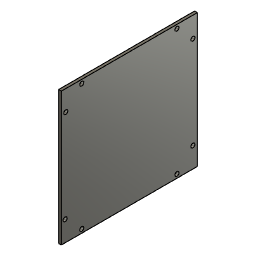
Сборка Cubesat 2.0 v6 (Autodesk Fusion 360 archive; units mm, degrees)
design "Боковые стенки Cubesat"
Autodesk Fusion 360 part; units mm, degrees
sketch "Sketch1" plane through (0, 0, 0) normal (1, 0, 0) x (0, 0, -1)
  line L0 (0, 0) -> (-100, 0)
  line L1 (-100, 0) -> (-100, 98)
  line L2 (-100, 98) -> (0, 98)
  line L3 (0, 98) -> (0, 0)
  dimension "d1" = 100
  dimension "d2" = 98
  constraint horizontal L0
  constraint vertical L1
  constraint horizontal L2
  constraint vertical L3
  constraint coincident L0.start L3.end
  measures "d1" distance of L0.start L0.end
  measures "d2" distance of L0.start L2.end
extrude "Extrude1" add sketch "Sketch1" against normal blind 2
extrude "Extrude2" add 1 faces at (0, 32.6667, 33.3333) along direction (1, 0, 0) blind 2
extrude "Extrude3" add 1 faces at (2, 32.6667, 33.3333) along direction (1, 0, 0) blind 1
sketch "Sketch2" plane through (3, 0, 0) normal (1, 0, 0) x (0, 0, -1)
  line L0 (-100, 98) -> (0, 98)
  line L1 (0, 98) -> (0, 0)
  line L2 (0, 0) -> (-100, 0)
  line L3 (-100, 0) -> (-100, 98)
  line L4 (-100, 98) -> (-85, 98)
  line L5 (-85, 98) -> (-85, 92.5)
  line L6 (-85, 92.5) -> (-100, 92.5)
  line L7 (-100, 92.5) -> (-100, 98)
  line L8 (-100, 98) -> (-93.5, 98)
  line L9 (-93.5, 98) -> (-93.5, 83)
  line L10 (0, 98) -> (-6.5, 98)
  line L11 (-6.5, 98) -> (-6.5, 83)
  line L12 (-6.5, 83) -> (0, 83)
  line L13 (0, 83) -> (0, 98)
  line L14 (0, 98) -> (-15, 98)
  line L15 (-15, 98) -> (-15, 92.5)
  line L16 (-15, 92.5) -> (0, 92.5)
  line L17 (0, 92.5) -> (0, 98)
  line L18 (0, 0) -> (-6.5, 0)
  line L19 (-6.5, 0) -> (-6.5, 15)
  line L20 (-6.5, 15) -> (0, 15)
  line L21 (0, 15) -> (0, 0)
  line L22 (0, 0) -> (-15, 0)
  line L23 (-15, 0) -> (-15, 5.5)
  line L24 (-15, 5.5) -> (0, 5.5)
  line L25 (0, 5.5) -> (0, 0)
  line L26 (-100, 0) -> (-85, 0)
  line L27 (-85, 0) -> (-85, 5.5)
  line L28 (-85, 5.5) -> (-100, 5.5)
  line L29 (-100, 5.5) -> (-100, 0)
  line L30 (-100, 0) -> (-94.5, 0)
  line L31 (-94.5, 0) -> (-94.5, 15)
  line L32 (-94.5, 15) -> (-100, 15)
  line L33 (-100, 15) -> (-100, 0)
  circle A0 centre (-85, 95.25) radius 1.5
  circle A1 centre (-97.25, 15) radius 1.5
  circle A2 centre (-85, 2.75) radius 1.5
  circle A3 centre (-15, 2.75) radius 1.5
  circle A4 centre (-3.25, 15) radius 1.5
  circle A5 centre (-3.25, 83) radius 1.5
  circle A6 centre (-15, 95.25) radius 1.5
  line L34 (-93.5, 83) -> (-100, 83)
  line L35 (-100, 83) -> (-100, 98)
  line L36 (-100, 98) -> (-93.5, 98)
  line L37 (-93.5, 98) -> (-93.5, 83)
  circle A7 centre (-96.75, 83) radius 1.5
  dimension "d53" = 15
  dimension "d54" = 5.5
  dimension "d55" = 6.5
  dimension "d57" = 6.5
  dimension "d58" = 15
  dimension "d59" = 15
  dimension "d60" = 5.5
  dimension "d61" = 6.5
  dimension "d62" = 15
  dimension "d63" = 5.5
  dimension "d64" = 15
  dimension "d65" = 5.5
  dimension "d66" = 15
  dimension "d67" = 100
  dimension "d68" = 98
  dimension "d69" = 5.5
  dimension "d70" = 15
  dimension "d71" = 3
  dimension "d73" = 3
  dimension "d74" = 3
  dimension "d75" = 3
  dimension "d76" = 3
  dimension "d77" = 3
  dimension "d78" = 3
  dimension "d81" = 15
  dimension "d83" = 3
  constraint horizontal L0
  constraint vertical L1
  constraint horizontal L2
  constraint vertical L3
  constraint coincident L1.end L2.start
  constraint horizontal L4
  constraint vertical L5
  constraint horizontal L6
  constraint vertical L7
  constraint horizontal L8
  constraint vertical L9
  constraint horizontal L10
  constraint vertical L11
  constraint horizontal L12
  constraint vertical L13
  constraint horizontal L14
  constraint vertical L15
  constraint horizontal L16
  constraint vertical L17
  constraint horizontal L18
  constraint vertical L19
  constraint horizontal L20
  constraint vertical L21
  constraint horizontal L22
  constraint vertical L23
  constraint horizontal L24
  constraint vertical L25
  constraint horizontal L26
  constraint vertical L27
  constraint horizontal L28
  constraint vertical L29
  constraint horizontal L30
  constraint vertical L31
  constraint horizontal L32
  constraint vertical L33
  constraint midpoint L5 A0.centre
  constraint midpoint L32 A1.centre
  constraint midpoint L27 A2.centre
  constraint midpoint L23 A3.centre
  constraint midpoint L20 A4.centre
  constraint midpoint L12 A5.centre
  constraint midpoint L15 A6.centre
  constraint horizontal L34
  constraint vertical L35
  constraint horizontal L36
  constraint vertical L37
  constraint midpoint L34 A7.centre
  measures "d53" distance of L0.start L4.end
  measures "d54" distance of L0.start L6.end
  measures "d55" distance of L0.start L8.end
  measures "d57" distance of L0.end L10.end
  measures "d58" distance of L0.end L12.end
  measures "d59" distance of L0.end L14.end
  measures "d60" distance of L0.end L16.end
  measures "d61" distance of L1.end L18.end
  measures "d62" distance of L1.end L20.end
  measures "d63" distance of L1.end L24.end
  measures "d64" distance of L2.end L26.end
  measures "d65" distance of L2.end L30.end
  measures "d66" distance of L2.end L32.end
  measures "d67" distance of L3 L13
  measures "d68" distance of L0 L2
  measures "d69" distance of L26 L28
  measures "d70" distance of L23 L25
  measures "d71" diameter of A0
  measures "d73" diameter of A1
  measures "d74" diameter of A2
  measures "d75" diameter of A3
  measures "d76" diameter of A4
  measures "d77" diameter of A5
  measures "d78" diameter of A6
  measures "d81" distance of L8 L34
  measures "d83" diameter of A7
extrude "Extrude9" cut sketch "Sketch2" against normal blind 20 contours L5 A0 | L5 A0 | L34 A7 | L34 A7 | L15 A6 | L15 A6 | L32 A1 | L32 A1 | L12 A5 | L12 A5 | L27 A2 | L27 A2 | L20 A4 | L20 A4 | L23 A3 | L23 A3
extrude "Extrude10" cut sketch "Sketch2" against normal blind 3 contours L0 L3 L4 L6 L7 L8 L9 L35 L36 L37 | L0 L4 L5 L6 L9 A0 L37 | L3 L6 L9 L34 L35 L37 A7 | L0 L1 L2 L3 L5 L6 L9 L11 L12 L15 L16 L19 L20 L23 L24 L27 L28 L31 L32 A0 A1 A2 A3 A4 A5 A6 L34 L37 A7 | L0 L11 L14 L15 L16 A6 | L3 L28 L31 L32 L33 A1 | L0 L1 L10 L11 L13 L14 L16 L17 | L2 L3 L26 L28 L29 L30 L31 L33 | L1 L11 L12 L13 L16 A5 | L2 L26 L27 L28 L31 A2 | L1 L19 L20 L21 L24 A4 | L2 L19 L22 L23 L24 A3 | L1 L2 L18 L19 L21 L22 L24 L25

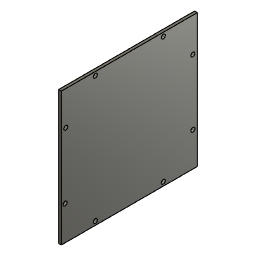
design "Боковые стенки Cubesat 2.0"
Autodesk Fusion 360 part; units mm, degrees
sketch "Sketch1" plane through (0, 0, 0) normal (1, 0, 0) x (0, 0, -1)
  line L0 (0, 0) -> (-100, 0)
  line L1 (-100, 0) -> (-100, 98)
  line L2 (-100, 98) -> (0, 98)
  line L3 (0, 98) -> (0, 0)
  dimension "d1" = 100
  dimension "d2" = 98
  constraint horizontal L0
  constraint vertical L1
  constraint horizontal L2
  constraint vertical L3
  constraint coincident L0.start L3.end
  measures "d1" distance of L0.start L0.end
  measures "d2" distance of L0.start L2.end
extrude "Extrude1" add sketch "Sketch1" against normal blind 2
extrude "Extrude2" add 1 faces at (0, 32.6667, 33.3333) along direction (1, 0, 0) blind 2
extrude "Extrude3" add 1 faces at (2, 32.6667, 33.3333) along direction (1, 0, 0) blind 1
sketch "Sketch2" plane through (3, 0, 0) normal (1, 0, 0) x (0, 0, -1)
  line L0 (-100, 98) -> (0, 98)
  line L1 (0, 98) -> (0, 0)
  line L2 (0, 0) -> (-100, 0)
  line L3 (-100, 0) -> (-100, 98)
  line L4 (-100, 98) -> (-75, 98)
  line L5 (-75, 98) -> (-75, 92.5)
  line L6 (-75, 92.5) -> (-100, 92.5)
  line L7 (-100, 92.5) -> (-100, 98)
  line L8 (-100, 98) -> (-93.5, 98)
  line L9 (-93.5, 98) -> (-93.5, 73)
  line L10 (0, 98) -> (-6.5, 98)
  line L11 (-6.5, 98) -> (-6.5, 73)
  line L12 (-6.5, 73) -> (0, 73)
  line L13 (0, 73) -> (0, 98)
  line L14 (0, 98) -> (-25, 98)
  line L15 (-25, 98) -> (-25, 92.5)
  line L16 (-25, 92.5) -> (0, 92.5)
  line L17 (0, 92.5) -> (0, 98)
  line L18 (0, 0) -> (-6.5, 0)
  line L19 (-6.5, 0) -> (-6.5, 25)
  line L20 (-6.5, 25) -> (0, 25)
  line L21 (0, 25) -> (0, 0)
  line L22 (0, 0) -> (-25, 0)
  line L23 (-25, 0) -> (-25, 5.5)
  line L24 (-25, 5.5) -> (0, 5.5)
  line L25 (0, 5.5) -> (0, 0)
  line L26 (-100, 0) -> (-75, 0)
  line L27 (-75, 0) -> (-75, 5.5)
  line L28 (-75, 5.5) -> (-100, 5.5)
  line L29 (-100, 5.5) -> (-100, 0)
  line L30 (-100, 0) -> (-94.5, 0)
  line L31 (-94.5, 0) -> (-94.5, 25)
  line L32 (-94.5, 25) -> (-100, 25)
  line L33 (-100, 25) -> (-100, 0)
  circle A0 centre (-75, 95.25) radius 1.5
  circle A1 centre (-97.25, 25) radius 1.5
  circle A2 centre (-75, 2.75) radius 1.5
  circle A3 centre (-25, 2.75) radius 1.5
  circle A4 centre (-3.25, 25) radius 1.5
  circle A5 centre (-3.25, 73) radius 1.5
  circle A6 centre (-25, 95.25) radius 1.5
  line L34 (-93.5, 73) -> (-100, 73)
  line L35 (-100, 73) -> (-100, 98)
  line L36 (-100, 98) -> (-93.5, 98)
  line L37 (-93.5, 98) -> (-93.5, 73)
  circle A7 centre (-96.75, 73) radius 1.5
  dimension "d53" = 25
  dimension "d54" = 5.5
  dimension "d55" = 6.5
  dimension "d57" = 6.5
  dimension "d58" = 25
  dimension "d59" = 25
  dimension "d60" = 5.5
  dimension "d61" = 6.5
  dimension "d62" = 25
  dimension "d63" = 5.5
  dimension "d64" = 25
  dimension "d65" = 5.5
  dimension "d66" = 25
  dimension "d67" = 100
  dimension "d68" = 98
  dimension "d69" = 5.5
  dimension "d70" = 25
  dimension "d71" = 3
  dimension "d73" = 3
  dimension "d74" = 3
  dimension "d75" = 3
  dimension "d76" = 3
  dimension "d77" = 3
  dimension "d78" = 3
  dimension "d81" = 25
  dimension "d83" = 3
  constraint horizontal L0
  constraint vertical L1
  constraint horizontal L2
  constraint vertical L3
  constraint coincident L1.end L2.start
  constraint horizontal L4
  constraint vertical L5
  constraint horizontal L6
  constraint vertical L7
  constraint horizontal L8
  constraint vertical L9
  constraint horizontal L10
  constraint vertical L11
  constraint horizontal L12
  constraint vertical L13
  constraint horizontal L14
  constraint vertical L15
  constraint horizontal L16
  constraint vertical L17
  constraint horizontal L18
  constraint vertical L19
  constraint horizontal L20
  constraint vertical L21
  constraint horizontal L22
  constraint vertical L23
  constraint horizontal L24
  constraint vertical L25
  constraint horizontal L26
  constraint vertical L27
  constraint horizontal L28
  constraint vertical L29
  constraint horizontal L30
  constraint vertical L31
  constraint horizontal L32
  constraint vertical L33
  constraint midpoint L5 A0.centre
  constraint midpoint L32 A1.centre
  constraint midpoint L27 A2.centre
  constraint midpoint L23 A3.centre
  constraint midpoint L20 A4.centre
  constraint midpoint L12 A5.centre
  constraint midpoint L15 A6.centre
  constraint horizontal L34
  constraint vertical L35
  constraint horizontal L36
  constraint vertical L37
  constraint midpoint L34 A7.centre
  measures "d53" distance of L0.start L4.end
  measures "d54" distance of L0.start L6.end
  measures "d55" distance of L0.start L8.end
  measures "d57" distance of L0.end L10.end
  measures "d58" distance of L0.end L12.end
  measures "d59" distance of L0.end L14.end
  measures "d60" distance of L0.end L16.end
  measures "d61" distance of L1.end L18.end
  measures "d62" distance of L1.end L20.end
  measures "d63" distance of L1.end L24.end
  measures "d64" distance of L2.end L26.end
  measures "d65" distance of L2.end L30.end
  measures "d66" distance of L2.end L32.end
  measures "d67" distance of L3 L13
  measures "d68" distance of L0 L2
  measures "d69" distance of L26 L28
  measures "d70" distance of L23 L25
  measures "d71" diameter of A0
  measures "d73" diameter of A1
  measures "d74" diameter of A2
  measures "d75" diameter of A3
  measures "d76" diameter of A4
  measures "d77" diameter of A5
  measures "d78" diameter of A6
  measures "d81" distance of L8 L34
  measures "d83" diameter of A7
extrude "Extrude9" cut sketch "Sketch2" against normal blind 20 contours L5 A0 | L5 A0 | L34 A7 | L34 A7 | L15 A6 | L15 A6 | L32 A1 | L32 A1 | L12 A5 | L12 A5 | L27 A2 | L27 A2 | L20 A4 | L20 A4 | L23 A3 | L23 A3
extrude "Extrude10" cut sketch "Sketch2" against normal blind 3 contours L0 L3 L4 L6 L7 L8 L9 L35 L36 L37 | L0 L4 L5 L6 L9 A0 L37 | L3 L6 L9 L34 L35 L37 A7 | L0 L1 L2 L3 L5 L6 L9 L11 L12 L15 L16 L19 L20 L23 L24 L27 L28 L31 L32 A0 A1 A2 A3 A4 A5 A6 L34 L37 A7 | L0 L11 L14 L15 L16 A6 | L3 L28 L31 L32 L33 A1 | L0 L1 L10 L11 L13 L14 L16 L17 | L2 L3 L26 L28 L29 L30 L31 L33 | L1 L11 L12 L13 L16 A5 | L2 L26 L27 L28 L31 A2 | L1 L19 L20 L21 L24 A4 | L2 L19 L22 L23 L24 A3 | L1 L2 L18 L19 L21 L22 L24 L25

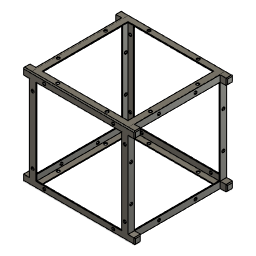
design "Cubesat 2.0"
Autodesk Fusion 360 part; units mm, degrees
sketch "Sketch1" plane through (0, 0, 0) normal (1, 0, 0) x (0, 0, -1)
  line L0 (0, 0) -> (-100, 0)
  line L1 (-100, 0) -> (-100, 100)
  line L2 (-100, 100) -> (0, 100)
  line L3 (0, 100) -> (0, 0)
  line L4 (-100, 100) -> (-93.5, 100)
  line L5 (-93.5, 100) -> (-93.5, 93.5)
  line L6 (-93.5, 93.5) -> (-100, 93.5)
  line L7 (-100, 93.5) -> (-100, 100)
  line L8 (0, 100) -> (-6.5, 100)
  line L9 (-6.5, 100) -> (-6.5, 93.5)
  line L10 (-6.5, 93.5) -> (0, 93.5)
  line L11 (0, 93.5) -> (0, 100)
  line L12 (-100, 0) -> (-93.5, 0)
  line L13 (-93.5, 0) -> (-93.5, 6.5)
  line L14 (-93.5, 6.5) -> (-100, 6.5)
  line L15 (-100, 6.5) -> (-100, 0)
  line L16 (0, 0) -> (-6.5, 0)
  line L17 (-6.5, 0) -> (-6.5, 6.5)
  line L18 (-6.5, 6.5) -> (0, 6.5)
  line L19 (0, 6.5) -> (0, 0)
  line L20 (-93.5, 93.5) -> (-6.5, 93.5)
  line L21 (-6.5, 93.5) -> (-6.5, 6.5)
  line L22 (-6.5, 6.5) -> (-93.5, 6.5)
  line L23 (-93.5, 6.5) -> (-93.5, 93.5)
  dimension "d1" = 100
  dimension "d2" = 100
  dimension "d3" = 6.5
  dimension "d4" = 6.5
  dimension "d5" = 6.5
  dimension "d6" = 6.5
  dimension "d7" = 6.5
  dimension "d8" = 6.5
  dimension "d9" = 6.5
  dimension "d10" = 6.5
  constraint horizontal L0
  constraint vertical L1
  constraint horizontal L2
  constraint vertical L3
  constraint coincident L0.start L3.end
  constraint horizontal L4
  constraint vertical L5
  constraint horizontal L6
  constraint vertical L7
  constraint horizontal L8
  constraint vertical L9
  constraint horizontal L10
  constraint vertical L11
  constraint horizontal L12
  constraint vertical L13
  constraint horizontal L14
  constraint vertical L15
  constraint horizontal L16
  constraint vertical L17
  constraint horizontal L18
  constraint vertical L19
  constraint horizontal L20
  constraint vertical L21
  constraint horizontal L22
  constraint vertical L23
  measures "d1" distance of L0.start L0.end
  measures "d2" distance of L0.start L2.end
  measures "d3" distance of L1.end L4.end
  measures "d4" distance of L1.end L6.end
  measures "d5" distance of L2.end L8.end
  measures "d6" distance of L2.end L10.end
  measures "d7" distance of L0.end L12.end
  measures "d8" distance of L0.end L14.end
  measures "d9" distance of L0.start L16.end
  measures "d10" distance of L0.start L18.end
extrude "Extrude1" add sketch "Sketch1" along normal blind 50 and the other way blind 50 contours L0 L3 L16 L17 L18 L19 | L0 L13 L17 L22 | L3 L10 L18 L21 | L0 L1 L12 L13 L14 L15 | L2 L3 L8 L9 L10 L11 | L1 L6 L14 L23 | L2 L5 L9 L20 | L1 L2 L4 L5 L6 L7
extrude "Extrude2" add sketch "Sketch1" along normal mid plane 113.5 contours L0 L3 L16 L17 L18 L19 | L0 L1 L12 L13 L14 L15 | L2 L3 L8 L9 L10 L11 | L1 L2 L4 L5 L6 L7
ref_plane "WorkPlane1" through (0, 50, 50) normal (0, 1, 0) x (0, 0, 1)
sketch "Sketch2" plane through (0, 50, 50) normal (0, 1, 0) x (1, 0, 0)
  line L0 (-50, -50) -> (50, -50)
  line L1 (50, -50) -> (50, 50)
  line L2 (50, 50) -> (-50, 50)
  line L3 (-50, 50) -> (-50, -50)
  line L4 (43.5, 43.5) -> (-43.5, 43.5)
  line L5 (-43.5, 43.5) -> (-43.5, -43.5)
  line L6 (-43.5, -43.5) -> (43.5, -43.5)
  line L7 (43.5, -43.5) -> (43.5, 43.5)
  line L8 (43.5, 43.5) -> (-43.5, -43.5) construction
  line L9 (-43.5, 43.5) -> (43.5, -43.5) construction
  dimension "d18" = 87
  dimension "d19" = 87
  dimension "d76" = 100
  dimension "d77" = 100
  dimension "d78" = 6.5
  dimension "d79" = 6.5
  constraint horizontal L0
  constraint vertical L1
  constraint horizontal L2
  constraint vertical L3
  constraint horizontal L4
  constraint perpendicular L4 L5
  constraint parallel L4 L6
  constraint parallel L5 L7
  constraint coincident L8 origin
  constraint coincident L9 origin
  measures "d18" distance of L5.end L6.end
  measures "d19" distance of L4.end L5.end
  measures "d76" distance of L1 L3
  measures "d77" distance of L0 L2
  measures "d78" distance of L1 L7
  measures "d79" distance of L0 L6
extrude "Extrude3" cut sketch "Sketch2" along normal mid plane 110 contours L4 L5 L6 L7
ref_plane "WorkPlane2" through (0, 50, 50) normal (0, 0, -1) x (0, 1, 0)
sketch "Sketch3" plane through (0, 50, 50) normal (0, 0, -1) x (1, 0, 0)
  line L0 (50, -50) -> (-50, -50)
  line L1 (-50, -50) -> (-50, 50)
  line L2 (-50, 50) -> (50, 50)
  line L3 (50, 50) -> (50, -50)
  line L4 (43.5, -43.5) -> (-43.5, -43.5)
  line L5 (-43.5, -43.5) -> (-43.5, 43.5)
  line L6 (-43.5, 43.5) -> (43.5, 43.5)
  line L7 (43.5, 43.5) -> (43.5, -43.5)
  line L8 (43.5, -43.5) -> (-43.5, 43.5) construction
  line L9 (-43.5, -43.5) -> (43.5, 43.5) construction
  dimension "d23" = 87
  dimension "d24" = 87
  dimension "d80" = 6.5
  dimension "d81" = 6.5
  dimension "d82" = 6.5
  dimension "d83" = 6.5
  constraint horizontal L0
  constraint vertical L1
  constraint horizontal L2
  constraint vertical L3
  constraint horizontal L4
  constraint perpendicular L4 L5
  constraint parallel L4 L6
  constraint parallel L5 L7
  constraint coincident L8 origin
  constraint coincident L9 origin
  measures "d23" distance of L5.end L6.end
  measures "d24" distance of L4.end L5.end
  measures "d80" distance of L2 L6
  measures "d81" distance of L1 L5
  measures "d82" distance of L3 L7
  measures "d83" distance of L0 L4
extrude "Extrude4" cut sketch "Sketch3" along normal mid plane 160 contours L4 L5 L6 L7
chamfer "Chamfer1" distance 0.8 angle 45 32 edges at (56.75, 100, 96.75) (56.75, 96.75, 100) (56.75, 96.75, 93.5) (56.75, 93.5, 96.75) (56.75, 6.5, 96.75) (56.75, 3.25, 93.5) (56.75, 0, 96.75) (56.75, 3.25, 100) (56.75, 0, 3.25) (56.75, 3.25, 6.5) (56.75, 6.5, 3.25) (56.75, 3.25, 0) (56.75, 100, 3.25) (56.75, 96.75, 6.5) (56.75, 93.5, 3.25) (56.75, 96.75, 0) (-56.75, 96.75, 0) (-56.75, 100, 3.25) (-56.75, 96.75, 6.5) (-56.75, 93.5, 3.25) (-56.75, 6.5, 3.25) (-56.75, 3.25, 0) (-56.75, 0, 3.25) (-56.75, 3.25, 6.5) (-56.75, 6.5, 96.75) (-56.75, 3.25, 93.5) (-56.75, 0, 96.75) (-56.75, 3.25, 100) (-56.75, 96.75, 93.5) (-56.75, 100, 96.75) (-56.75, 96.75, 100) (-56.75, 93.5, 96.75)
fillet "Fillet1" radius 1 4 edges at (0, 100, 100) (0, 100, 0) (0, 0, 100) (0, 0, 0)
ref_plane "WorkPlane3" through (0, 96.75, 3.25) normal (-1, 0, 0) x (0, 0, 1)
sketch "Sketch4" plane through (0, 96.75, 3.25) normal (-1, 0, 0) x (0, 0, -1)
  line L0 (2.45, 91.05) -> (-2.45, 91.05) construction
  line L1 (-2.45, 91.05) -> (-2.45, 95.95) construction
  line L2 (-2.45, 95.95) -> (2.45, 95.95) construction
  line L3 (2.45, 95.95) -> (2.45, 91.05) construction
  line L4 (-95.95, 95.95) -> (-91.05, 95.95) construction
  line L5 (-91.05, 95.95) -> (-91.05, 91.05) construction
  line L6 (-91.05, 91.05) -> (-95.95, 91.05) construction
  line L7 (-95.95, 91.05) -> (-95.95, 95.95) construction
  line L8 (-95.95, 2.45) -> (-91.05, 2.45) construction
  line L9 (-91.05, 2.45) -> (-91.05, -2.45) construction
  line L10 (-91.05, -2.45) -> (-95.95, -2.45) construction
  line L11 (-95.95, -2.45) -> (-95.95, 2.45) construction
  line L12 (-2.45, 2.45) -> (2.45, 2.45) construction
  line L13 (2.45, 2.45) -> (2.45, -2.45) construction
  line L14 (2.45, -2.45) -> (-2.45, -2.45) construction
  line L15 (-2.45, -2.45) -> (-2.45, 2.45) construction
  line L16 (2.45, 95.95) -> (-2.45, 91.05) construction
  line L17 (2.45, 91.05) -> (-2.45, 95.95) construction
  line L18 (-91.05, 2.45) -> (-95.95, -2.45) construction
  line L19 (-91.05, -2.45) -> (-95.95, 2.45) construction
  line L20 (0, 93.5) -> (-93.5, 93.5)
  line L21 (-93.5, 93.5) -> (-93.5, 0)
  line L22 (-93.5, 0) -> (0, 0)
  line L23 (0, 0) -> (0, 93.5)
  constraint coincident L2.end L3.start
  constraint coincident L0.end L1.start
  constraint coincident L0.start L3.end
  constraint coincident L1.end L2.start
  constraint coincident L8.end L9.start
  constraint coincident L10.end L11.start
  constraint coincident L9.end L10.start
  constraint coincident L8.start L11.end
  constraint horizontal L20
  constraint vertical L21
  constraint horizontal L22
  constraint vertical L23
  constraint midpoint L18 L21.end
  constraint midpoint L17 L20.start
extrude "Extrude5" cut sketch "Sketch4" along normal mid plane 98
sketch "Sketch5" plane through (0, 0, 3.25) normal (0, 0, 1) x (1, 0, 0)
  line L0 (43.5, 6.5) -> (-43.5, 6.5)
  line L1 (-43.5, 6.5) -> (-43.5, 93.5)
  line L2 (-43.5, 93.5) -> (43.5, 93.5)
  line L3 (43.5, 93.5) -> (43.5, 6.5)
  line L4 (-49, 3.25) -> (49, 3.25)
  line L5 (49, 3.25) -> (49, 96.75)
  line L6 (49, 96.75) -> (-49, 96.75)
  line L7 (-49, 96.75) -> (-49, 3.25)
  line L8 (49, 0.75) -> (-49, 0.75)
  line L9 (49, 0.75) -> (49, 99.25)
  line L10 (49, 99.25) -> (-49, 99.25)
  line L11 (-49, 99.25) -> (-49, 0.75)
  dimension "d32" = 2.5
  dimension "d33" = 2.5
  constraint perpendicular L7 L8
  constraint perpendicular L8 L9
  constraint perpendicular L9 L10
  constraint coincident L5 L8.start
  constraint coincident L6.end L11
  constraint vertical L11
  measures "d32" distance of L4 L8
  measures "d33" distance of L6 L10
extrude "Extrude6" cut sketch "Sketch5" along normal blind 95.75 and the other way blind 2.25
sketch "Sketch6" plane through (0, 0, 0) normal (1, 0, 0) x (0, 0, -1)
sketch "Sketch7" plane through (50, 0, 0) normal (1, 0, 0) x (0, 0, -1)
  line L0 (-6.5, 93.5) -> (-6.5, 100)
  line L1 (-6.5, 100) -> (-93.5, 100)
  line L2 (-93.5, 100) -> (-93.5, 93.5)
  line L3 (-93.5, 93.5) -> (-6.5, 93.5)
  line L4 (-93.5, 100) -> (-68.5, 100)
  line L5 (-68.5, 100) -> (-68.5, 93.5)
  line L6 (-68.5, 93.5) -> (-93.5, 93.5)
  line L7 (-93.5, 93.5) -> (-93.5, 100)
  line L8 (-6.5, 100) -> (-31.5, 100)
  line L9 (-31.5, 100) -> (-31.5, 93.5)
  line L10 (-31.5, 93.5) -> (-6.5, 93.5)
  line L11 (-6.5, 93.5) -> (-6.5, 100)
  circle A0 centre (-68.5, 96.75) radius 1.5
  circle A1 centre (-31.5, 96.75) radius 1.5
  line L12 (-93.5, 93.5) -> (-100, 93.5)
  line L13 (-100, 93.5) -> (-100, 6.5)
  line L14 (-100, 6.5) -> (-93.5, 6.5)
  line L15 (-93.5, 6.5) -> (-93.5, 93.5)
  line L16 (-100, 6.5) -> (-93.5, 6.5)
  line L17 (-93.5, 6.5) -> (-93.5, 31.5)
  line L18 (-93.5, 31.5) -> (-100, 31.5)
  line L19 (-100, 31.5) -> (-100, 6.5)
  line L20 (-100, 93.5) -> (-93.5, 93.5)
  line L21 (-93.5, 93.5) -> (-93.5, 68.5)
  line L22 (-93.5, 68.5) -> (-100, 68.5)
  line L23 (-100, 68.5) -> (-100, 93.5)
  line L24 (-93.5, 6.5) -> (-68.5, 6.5)
  line L25 (-68.5, 6.5) -> (-68.5, 0)
  line L26 (-68.5, 0) -> (-93.5, 0)
  line L27 (-93.5, 0) -> (-93.5, 6.5)
  line L28 (-6.4996, 6.5) -> (-31.4996, 6.5)
  line L29 (-31.4996, 6.5) -> (-31.4996, 0)
  line L30 (-31.4996, 0) -> (-6.4996, 0)
  line L31 (-6.4996, 0) -> (-6.4996, 6.5)
  line L32 (-6.4996, 6.5) -> (0, 6.5)
  line L33 (0, 6.5) -> (0, 31.5)
  line L34 (0, 31.5) -> (-6.4996, 31.5)
  line L35 (-6.4996, 31.5) -> (-6.4996, 6.5)
  line L36 (-6.5, 93.5) -> (0, 93.5)
  line L37 (0, 93.5) -> (0, 68.5)
  line L38 (0, 68.5) -> (-6.5, 68.5)
  line L39 (-6.5, 68.5) -> (-6.5, 93.5)
  circle A2 centre (-96.75, 68.5) radius 1.5
  circle A3 centre (-96.75, 31.5) radius 1.5
  circle A4 centre (-68.5, 3.25) radius 1.5
  circle A5 centre (-31.4996, 3.25) radius 1.5
  circle A6 centre (-3.2498, 31.5) radius 1.5
  circle A7 centre (-3.25, 68.5) radius 1.5
  point P0 (-100, 93.5)
  point P1 (-6.5, 6.5)
  dimension "d36" = 25
  dimension "d37" = 25
  dimension "d38" = 3
  dimension "d39" = 3
  dimension "d40" = 3.25
  dimension "d41" = 3.25
  dimension "d42" = 25
  dimension "d43" = 25
  dimension "d44" = 25
  dimension "d45" = 25
  dimension "d46" = 25
  dimension "d47" = 6.5
  dimension "d48" = 25
  dimension "d49" = 3
  dimension "d50" = 3
  dimension "d51" = 3
  dimension "d52" = 3
  dimension "d53" = 3
  dimension "d54" = 3
  dimension "d55" = 3.25
  dimension "d56" = 87
  dimension "d57" = 3.25
  dimension "d58" = 3.25
  dimension "d59" = 3.25
  dimension "d60" = 37.0004
  dimension "d61" = 3.2498
  constraint horizontal L4
  constraint vertical L5
  constraint horizontal L6
  constraint vertical L7
  constraint coincident L1.end L2.start
  constraint horizontal L8
  constraint vertical L9
  constraint horizontal L10
  constraint vertical L11
  constraint coincident L0.end L1.start
  constraint midpoint L5 A0.centre
  constraint midpoint L9 A1.centre
  constraint horizontal L12
  constraint vertical L13
  constraint horizontal L14
  constraint vertical L15
  constraint horizontal L16
  constraint vertical L17
  constraint horizontal L18
  constraint vertical L19
  constraint horizontal L20
  constraint vertical L21
  constraint horizontal L22
  constraint vertical L23
  constraint horizontal L24
  constraint vertical L25
  constraint horizontal L26
  constraint vertical L27
  constraint horizontal L28
  constraint vertical L29
  constraint horizontal L30
  constraint vertical L31
  constraint horizontal L32
  constraint vertical L33
  constraint horizontal L34
  constraint vertical L35
  constraint horizontal L36
  constraint vertical L37
  constraint horizontal L38
  constraint vertical L39
  constraint midpoint L22 A2.centre
  constraint midpoint L18 A3.centre
  constraint midpoint L25 A4.centre
  constraint midpoint L29 A5.centre
  constraint midpoint L34 A6.centre
  constraint midpoint L38 A7.centre
  constraint coincident L13 P0
  constraint coincident L28 P1
  measures "d36" distance of L1.end L4.end
  measures "d37" distance of L0.end L8.end
  measures "d38" diameter of A0
  measures "d39" diameter of A1
  measures "d40" distance of L4 A0.centre
  measures "d41" distance of L10 A1.centre
  measures "d42" distance of L13.end L18.end
  measures "d43" distance of P0 L22.end
  measures "d44" distance of L14.end L24.end
  measures "d45" distance of L28.start L28.end
  measures "d46" distance of L28.start L34.end
  measures "d47" distance of L0.start L36.end
  measures "d48" distance of L0.start L38.end
  measures "d49" diameter of A2
  measures "d50" diameter of A3
  measures "d51" diameter of A4
  measures "d52" diameter of A5
  measures "d53" diameter of A6
  measures "d54" diameter of A7
  measures "d55" distance of L21 A2.centre
  measures "d56" distance of P0 L13.end
  measures "d57" distance of L13 A3.centre
  measures "d58" distance of L24 A4.centre
  measures "d59" distance of L28 A5.centre
  measures "d60" distance of A4.centre A5.centre
  measures "d61" distance of L35 A6.centre
extrude "Extrude7" cut sketch "Sketch7" against normal blind 120 contours L9 A1 | L9 A1 | L38 A7 | L38 A7 | L5 A0 | L5 A0 | L22 A2 | L22 A2 | L18 A3 | L18 A3 | L25 A4 | L25 A4 | L29 A5 | L29 A5 | L34 A6 | L34 A6
sketch "Sketch8" plane through (0, 0, 0) normal (0, 0, -1) x (-1, 0, 0)
  line L0 (-55.95, 1) -> (55.95, 1)
  line L1 (55.95, 1) -> (55.95, 6.5)
  line L2 (55.95, 6.5) -> (50, 6.5)
  line L3 (50, 6.5) -> (50, 93.5)
  line L4 (50, 93.5) -> (55.95, 93.5)
  line L5 (55.95, 93.5) -> (55.95, 99)
  line L6 (55.95, 99) -> (-55.95, 99)
  line L7 (-55.95, 99) -> (-55.95, 93.5)
  line L8 (-55.95, 93.5) -> (-50, 93.5)
  line L9 (-50, 93.5) -> (-50, 6.5)
  line L10 (-50, 6.5) -> (-55.95, 6.5)
  line L11 (-55.95, 6.5) -> (-55.95, 1)
  line L12 (-43.5, 6.5) -> (-43.5, 93.5)
  line L13 (-43.5, 93.5) -> (43.5, 93.5)
  line L14 (43.5, 93.5) -> (43.5, 6.5)
  line L15 (43.5, 6.5) -> (-43.5, 6.5)
  line L16 (-50, 93.5) -> (-35, 93.5)
  line L17 (-35, 93.5) -> (-35, 99)
  line L18 (-35, 99) -> (-50, 99)
  line L19 (-50, 99) -> (-50, 93.5)
  line L20 (-50, 99) -> (-43.5, 99)
  line L21 (-43.5, 99) -> (-43.5, 84)
  line L22 (-43.5, 84) -> (-50, 84)
  line L23 (-50, 84) -> (-50, 99)
  line L24 (50, 93.5) -> (35, 93.5)
  line L25 (35, 93.5) -> (35, 99)
  line L26 (35, 99) -> (50, 99)
  line L27 (50, 99) -> (50, 93.5)
  line L28 (50, 99) -> (43.5, 99)
  line L29 (43.5, 99) -> (43.5, 84)
  line L30 (43.5, 84) -> (50, 84)
  line L31 (50, 84) -> (50, 99)
  line L32 (50, 6.5) -> (35, 6.5)
  line L33 (35, 6.5) -> (35, 1)
  line L34 (35, 1) -> (50, 1)
  line L35 (50, 1) -> (50, 6.5)
  line L36 (50, 1) -> (43.5, 1)
  line L37 (43.5, 1) -> (43.5, 16)
  line L38 (43.5, 16) -> (50, 16)
  line L39 (50, 16) -> (50, 1)
  line L40 (-50, 1) -> (-43.5, 1)
  line L41 (-43.5, 1) -> (-43.5, 16)
  line L42 (-43.5, 16) -> (-50, 16)
  line L43 (-50, 16) -> (-50, 1)
  line L44 (-50, 6.5) -> (-35, 6.5)
  line L45 (-35, 6.5) -> (-35, 1)
  line L46 (-35, 1) -> (-50, 1)
  line L47 (-50, 1) -> (-50, 6.5)
  circle A0 centre (35, 3.75) radius 1.5
  circle A1 centre (-35, 3.75) radius 1.5
  circle A2 centre (-46.75, 16) radius 1.5
  circle A3 centre (-46.75, 84) radius 1.5
  circle A4 centre (-35, 96.25) radius 1.5
  circle A5 centre (35, 96.25) radius 1.5
  circle A6 centre (46.75, 84) radius 1.5
  circle A7 centre (46.75, 16) radius 1.5
  dimension "d66" = 15
  dimension "d67" = 15
  dimension "d68" = 5.5
  dimension "d69" = 6.5
  dimension "d70" = 15
  dimension "d71" = 15
  dimension "d72" = 6.5
  dimension "d73" = 5.5
  dimension "d74" = 15
  dimension "d75" = 15
  dimension "d84" = 5.5
  dimension "d85" = 15
  dimension "d86" = 15
  dimension "d87" = 3
  dimension "d88" = 3
  dimension "d89" = 3
  dimension "d90" = 3
  dimension "d91" = 3
  dimension "d92" = 3
  dimension "d93" = 3
  dimension "d94" = 3
  dimension "d95" = 2.75
  dimension "d96" = 3.25
  dimension "d97" = 8.5
  constraint horizontal L16
  constraint vertical L17
  constraint horizontal L18
  constraint vertical L19
  constraint coincident L8.end L9.start
  constraint horizontal L20
  constraint vertical L21
  constraint horizontal L22
  constraint vertical L23
  constraint horizontal L24
  constraint vertical L25
  constraint horizontal L26
  constraint vertical L27
  constraint coincident L3.end L4.start
  constraint horizontal L28
  constraint vertical L29
  constraint horizontal L30
  constraint vertical L31
  constraint horizontal L32
  constraint vertical L33
  constraint horizontal L34
  constraint vertical L35
  constraint coincident L2.end L3.start
  constraint horizontal L36
  constraint vertical L37
  constraint horizontal L38
  constraint vertical L39
  constraint coincident L14 L37.end
  constraint horizontal L40
  constraint vertical L41
  constraint horizontal L42
  constraint vertical L43
  constraint coincident L0 L40.start
  constraint horizontal L44
  constraint vertical L45
  constraint horizontal L46
  constraint vertical L47
  constraint coincident L9.end L10.start
  constraint midpoint L33 A0.centre
  constraint midpoint L45 A1.centre
  constraint midpoint L42 A2.centre
  constraint midpoint L22 A3.centre
  constraint midpoint L17 A4.centre
  constraint midpoint L25 A5.centre
  constraint midpoint L30 A6.centre
  constraint midpoint L38 A7.centre
  measures "d66" distance of L8.end L16.end
  measures "d67" distance of L18.end L22.end
  measures "d68" distance of L16 L18
  measures "d69" distance of L19 L21
  measures "d70" distance of L3.end L24.end
  measures "d71" distance of L26.end L30.end
  measures "d72" distance of L29 L31
  measures "d73" distance of L24 L26
  measures "d74" distance of L2.end L32.end
  measures "d75" distance of L34.end L38.end
  measures "d84" distance of L32 L34
  measures "d85" distance of L40.start L42.end
  measures "d86" distance of L9.end L44.end
  measures "d87" diameter of A0
  measures "d88" diameter of A1
  measures "d89" diameter of A2
  measures "d90" diameter of A3
  measures "d91" diameter of A4
  measures "d92" diameter of A5
  measures "d93" diameter of A6
  measures "d94" diameter of A7
  measures "d95" distance of L46 A1.centre
  measures "d96" distance of L41 A2.centre
  measures "d97" distance of L41 A1.centre
extrude "Extrude8" cut sketch "Sketch8" against normal blind 160 contours L45 A1 | L45 A1 | L42 A2 | L42 A2 | L33 A0 | L33 A0 | L22 A3 | L22 A3 | L38 A7 | L38 A7 | L17 A4 | L17 A4 | L30 A6 | L30 A6 | L25 A5 | L25 A5
sketch "Sketch9" plane through (0, 0, 0) normal (0, 0, -1) x (-1, 0, 0)
  circle A0 centre (-46.75, 84) radius 1.5
  circle A1 centre (46.75, 16) radius 1.5
  circle A2 centre (46.75, 84) radius 1.5
  circle A3 centre (-46.75, 16) radius 1.5
  circle A4 centre (-35, 96.25) radius 1.5
  circle A5 centre (35, 3.75) radius 1.5
  circle A6 centre (35, 96.25) radius 1.5
  circle A7 centre (-35, 3.75) radius 1.5
  line L0 (-55.95, 1) -> (55.95, 1)
  line L1 (55.95, 1) -> (55.95, 6.5)
  line L2 (55.95, 6.5) -> (50, 6.5)
  line L3 (50, 6.5) -> (50, 93.5)
  line L4 (50, 93.5) -> (55.95, 93.5)
  line L5 (55.95, 93.5) -> (55.95, 99)
  line L6 (55.95, 99) -> (-55.95, 99)
  line L7 (-55.95, 99) -> (-55.95, 93.5)
  line L8 (-55.95, 93.5) -> (-50, 93.5)
  line L9 (-50, 93.5) -> (-50, 6.5)
  line L10 (-50, 6.5) -> (-55.95, 6.5)
  line L11 (-55.95, 6.5) -> (-55.95, 1)
  line L12 (-43.5, 6.5) -> (-43.5, 93.5)
  line L13 (-43.5, 93.5) -> (43.5, 93.5)
  line L14 (43.5, 93.5) -> (43.5, 6.5)
  line L15 (43.5, 6.5) -> (-43.5, 6.5)
sketch "Sketch11" plane through (0, 100, 0) normal (0, 1, 0) x (-1, 0, 0)
  line L0 (-43.5, 93.5) -> (43.5, 93.5)
  line L1 (43.5, 93.5) -> (43.5, 6.5)
  line L2 (43.5, 6.5) -> (-43.5, 6.5)
  line L3 (-43.5, 6.5) -> (-43.5, 93.5)
  line L4 (-55.95, 1) -> (55.95, 1)
  line L5 (55.95, 1) -> (55.95, 6.5)
  line L6 (55.95, 6.5) -> (50, 6.5)
  line L7 (50, 6.5) -> (50, 93.5)
  line L8 (50, 93.5) -> (55.95, 93.5)
  line L9 (55.95, 93.5) -> (55.95, 99)
  line L10 (55.95, 99) -> (-55.95, 99)
  line L11 (-55.95, 99) -> (-55.95, 93.5)
  line L12 (-55.95, 93.5) -> (-50, 93.5)
  line L13 (-50, 93.5) -> (-50, 6.5)
  line L14 (-50, 6.5) -> (-55.95, 6.5)
  line L15 (-55.95, 6.5) -> (-55.95, 1)
  line L16 (-50, 1) -> (50, 1)
  line L17 (50, 1) -> (50, 99)
  line L18 (50, 99) -> (-50, 99)
  line L19 (-50, 99) -> (-50, 1)
  line L20 (50, 1) -> (25, 1)
  line L21 (25, 1) -> (25, 6.5)
  line L22 (25, 6.5) -> (50, 6.5)
  line L23 (50, 6.5) -> (50, 1)
  line L24 (50, 1) -> (43.5, 1)
  line L25 (43.5, 1) -> (43.5, 26)
  line L26 (43.5, 26) -> (50, 26)
  line L27 (50, 26) -> (50, 1)
  line L28 (-50, 1) -> (-25, 1)
  line L29 (-25, 1) -> (-25, 6.5)
  line L30 (-25, 6.5) -> (-50, 6.5)
  line L31 (-50, 6.5) -> (-50, 1)
  line L32 (-50, 1) -> (-43.5, 1)
  line L33 (-43.5, 1) -> (-43.5, 26)
  line L34 (-43.5, 26) -> (-50, 26)
  line L35 (-50, 26) -> (-50, 1)
  line L36 (-50, 99) -> (-43.5, 99)
  line L37 (-43.5, 99) -> (-43.5, 74)
  line L38 (-43.5, 74) -> (-50, 74)
  line L39 (-50, 74) -> (-50, 99)
  line L40 (-50, 99) -> (-25, 99)
  line L41 (-25, 99) -> (-25, 93.5)
  line L42 (-25, 93.5) -> (-50, 93.5)
  line L43 (-50, 93.5) -> (-50, 99)
  line L44 (50, 99) -> (25, 99)
  line L45 (25, 99) -> (25, 93.5)
  line L46 (25, 93.5) -> (50, 93.5)
  line L47 (50, 93.5) -> (50, 99)
  line L48 (50, 99) -> (43.5, 99)
  line L49 (43.5, 99) -> (43.5, 74)
  line L50 (43.5, 74) -> (50, 74)
  line L51 (50, 74) -> (50, 99)
  circle A0 centre (25, 3.75) radius 1.5
  circle A1 centre (46.75, 26) radius 1.5
  circle A2 centre (-25, 3.75) radius 1.5
  circle A3 centre (-46.75, 26) radius 1.5
  circle A4 centre (-46.75, 74) radius 1.5
  circle A5 centre (-25, 96.25) radius 1.5
  circle A6 centre (25, 96.25) radius 1.5
  circle A7 centre (46.75, 74) radius 1.5
  dimension "d109" = 100
  dimension "d110" = 98
  dimension "d111" = 6.5
  dimension "d112" = 25
  dimension "d113" = 5.5
  dimension "d114" = 25
  dimension "d115" = 25
  dimension "d116" = 5.5
  dimension "d117" = 25
  dimension "d118" = 6.5
  dimension "d119" = 25
  dimension "d120" = 25
  dimension "d121" = 25
  dimension "d122" = 5.5
  dimension "d123" = 25
  dimension "d124" = 6.5
  dimension "d125" = 6.5
  dimension "d126" = 5.5
  dimension "d127" = 6.5
  dimension "d128" = 3
  dimension "d129" = 3
  dimension "d130" = 3
  dimension "d131" = 3
  dimension "d132" = 3
  dimension "d133" = 3
  dimension "d134" = 3
  dimension "d135" = 3
  constraint horizontal L16
  constraint vertical L17
  constraint horizontal L18
  constraint vertical L19
  constraint coincident L4 L16.start
  constraint horizontal L20
  constraint vertical L21
  constraint horizontal L22
  constraint vertical L23
  constraint horizontal L24
  constraint vertical L25
  constraint horizontal L26
  constraint vertical L27
  constraint horizontal L28
  constraint vertical L29
  constraint horizontal L30
  constraint vertical L31
  constraint horizontal L32
  constraint vertical L33
  constraint horizontal L34
  constraint vertical L35
  constraint horizontal L36
  constraint vertical L37
  constraint horizontal L38
  constraint vertical L39
  constraint horizontal L40
  constraint vertical L41
  constraint horizontal L42
  constraint vertical L43
  constraint horizontal L44
  constraint vertical L45
  constraint horizontal L46
  constraint vertical L47
  constraint horizontal L48
  constraint vertical L49
  constraint horizontal L50
  constraint vertical L51
  constraint midpoint L21 A0.centre
  constraint midpoint L26 A1.centre
  constraint midpoint L29 A2.centre
  constraint midpoint L34 A3.centre
  constraint midpoint L38 A4.centre
  constraint midpoint L41 A5.centre
  constraint midpoint L45 A6.centre
  constraint midpoint L50 A7.centre
  measures "d109" distance of L16.start L16.end
  measures "d110" distance of L16.start L18.end
  measures "d111" distance of L3 L19
  measures "d112" distance of L16.end L20.end
  measures "d113" distance of L16.end L6.end
  measures "d114" distance of L16.end L26.end
  measures "d115" distance of L16.start L28.end
  measures "d116" distance of L16.start L13.end
  measures "d117" distance of L16.start L34.end
  measures "d118" distance of L33.end L34.end
  measures "d119" distance of L18.end L38.end
  measures "d120" distance of L18.end L40.end
  measures "d121" distance of L17.end L44.end
  measures "d122" distance of L44.end L45.end
  measures "d123" distance of L17.end L50.end
  measures "d124" distance of L25 L27
  measures "d125" distance of L19 L37
  measures "d126" distance of L18 L42
  measures "d127" distance of L17 L49
  measures "d128" diameter of A0
  measures "d129" diameter of A1
  measures "d130" diameter of A2
  measures "d131" diameter of A3
  measures "d132" diameter of A4
  measures "d133" diameter of A5
  measures "d134" diameter of A6
  measures "d135" diameter of A7
extrude "Extrude9" cut sketch "Sketch11" against normal blind 120 contours L41 A5 | L41 A5 | L38 A4 | L38 A4 | L45 A6 | L45 A6 | L34 A3 | L34 A3 | L50 A7 | L50 A7 | L29 A2 | L29 A2 | L26 A1 | L26 A1 | L21 A0 | L21 A0

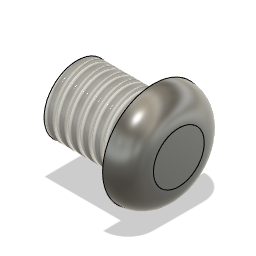
design "Болт M4"
Autodesk Fusion 360 part; units mm, degrees
sketch "Sketch1" plane through (0, 0, 0) normal (1, 0, 0) x (0, 0, -1)
  circle A0 centre (0, 0) radius 1.5
  dimension "d1" = 3
  constraint coincident A0.centre origin
  measures "d1" diameter of A0
extrude "Extrude1" add sketch "Sketch1" along normal blind 4.5
sketch "Sketch2" plane through (4.5, 0, 0) normal (1, 0, 0) x (0, 0, -1)
  circle A0 centre (0, 0) radius 1.5
  circle A1 centre (0, 0) radius 3
  dimension "d4" = 6
  constraint concentric A0 A1
  measures "d4" diameter of A1
extrude "Extrude2" add sketch "Sketch2" along normal blind 1.5 contours A0 | A1
fillet "Fillet1" radius 1.5 1 edges at (6, -1.0848, 2.797)
thread "Thread1" "ISO Metric profile 4.0 M4x0.7 6g" major diameter 3.908 minor diameter 3.111 pitch 0.7 angle 60 resizes the face on face at (3, -0.0748, -1.4981)

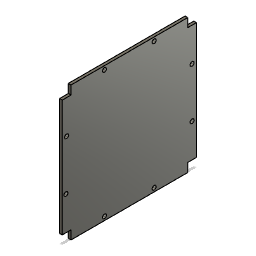
design "Боковые стенки Cubesatb 3.0"
Autodesk Fusion 360 part; units mm, degrees
sketch "Sketch1" plane through (0, 0, 0) normal (1, 0, 0) x (0, 0, -1)
  line L0 (0, 0) -> (-100, 0)
  line L1 (-100, 0) -> (-100, 100)
  line L2 (-100, 100) -> (0, 100)
  line L3 (0, 100) -> (0, 0)
  dimension "d1" = 100
  dimension "d2" = 100
  constraint horizontal L0
  constraint vertical L1
  constraint horizontal L2
  constraint vertical L3
  constraint coincident L0.start L3.end
  measures "d1" distance of L0.start L0.end
  measures "d2" distance of L0.start L2.end
extrude "Extrude1" add sketch "Sketch1" against normal blind 2
extrude "Extrude2" add 1 faces at (0, 33.3333, 33.3333) along direction (1, 0, 0) blind 2
extrude "Extrude3" add 1 faces at (2, 33.3333, 33.3333) along direction (1, 0, 0) blind 1
sketch "Sketch2" plane through (3, 0, 0) normal (1, 0, 0) x (0, 0, -1)
  line L0 (-100, 100) -> (0, 100)
  line L1 (0, 100) -> (0, 0)
  line L2 (0, 0) -> (-100, 0)
  line L3 (-100, 0) -> (-100, 100)
  line L4 (-100, 100) -> (-68.5, 100)
  line L5 (-68.5, 100) -> (-68.5, 94.5)
  line L6 (-68.5, 94.5) -> (-100, 94.5)
  line L7 (-100, 94.5) -> (-100, 100)
  line L8 (-100, 100) -> (-93.5, 100)
  line L9 (-93.5, 100) -> (-93.5, 68.5)
  line L10 (0, 100) -> (-6.5, 100)
  line L11 (-6.5, 100) -> (-6.5, 68.5)
  line L12 (-6.5, 68.5) -> (0, 68.5)
  line L13 (0, 68.5) -> (0, 100)
  line L14 (0, 100) -> (-31.5, 100)
  line L15 (-31.5, 100) -> (-31.5, 94.5)
  line L16 (-31.5, 94.5) -> (0, 94.5)
  line L17 (0, 94.5) -> (0, 100)
  line L18 (0, 0) -> (-6.5, 0)
  line L19 (-6.5, 0) -> (-6.5, 31.5)
  line L20 (-6.5, 31.5) -> (0, 31.5)
  line L21 (0, 31.5) -> (0, 0)
  line L22 (0, 0) -> (-31.5, 0)
  line L23 (-31.5, 0) -> (-31.5, 5.5)
  line L24 (-31.5, 5.5) -> (0, 5.5)
  line L25 (0, 5.5) -> (0, 0)
  line L26 (-100, 0) -> (-68.5, 0)
  line L27 (-68.5, 0) -> (-68.5, 5.5)
  line L28 (-68.5, 5.5) -> (-100, 5.5)
  line L29 (-100, 5.5) -> (-100, 0)
  line L30 (-100, 0) -> (-94.5, 0)
  line L31 (-94.5, 0) -> (-94.5, 31.5)
  line L32 (-94.5, 31.5) -> (-100, 31.5)
  line L33 (-100, 31.5) -> (-100, 0)
  circle A0 centre (-68.5, 97.25) radius 1.5
  circle A1 centre (-97.25, 31.5) radius 1.5
  circle A2 centre (-68.5, 2.75) radius 1.5
  circle A3 centre (-31.5, 2.75) radius 1.5
  circle A4 centre (-3.25, 31.5) radius 1.5
  circle A5 centre (-3.25, 68.5) radius 1.5
  circle A6 centre (-31.5, 97.25) radius 1.5
  line L34 (-93.5, 68.5) -> (-100, 68.5)
  line L35 (-100, 68.5) -> (-100, 100)
  line L36 (-100, 100) -> (-93.5, 100)
  line L37 (-93.5, 100) -> (-93.5, 68.5)
  circle A7 centre (-96.75, 68.5) radius 1.5
  line L38 (-100, 100) -> (-93.5, 100)
  line L39 (-93.5, 100) -> (-93.5, 93.5)
  line L40 (-93.5, 93.5) -> (-100, 93.5)
  line L41 (-100, 93.5) -> (-100, 100)
  line L42 (-100, 0) -> (-93.5, 0)
  line L43 (-93.5, 0) -> (-93.5, 6.5)
  line L44 (-93.5, 6.5) -> (-100, 6.5)
  line L45 (-100, 6.5) -> (-100, 0)
  line L46 (0, 0) -> (-6.5, 0)
  line L47 (-6.5, 0) -> (-6.5, 6.5)
  line L48 (-6.5, 6.5) -> (0, 6.5)
  line L49 (0, 6.5) -> (0, 0)
  line L50 (0, 100) -> (-6.5, 100)
  line L51 (-6.5, 100) -> (-6.5, 93.5)
  line L52 (-6.5, 93.5) -> (0, 93.5)
  line L53 (0, 93.5) -> (0, 100)
  dimension "d53" = 31.5
  dimension "d54" = 5.5
  dimension "d55" = 6.5
  dimension "d57" = 6.5
  dimension "d58" = 31.5
  dimension "d59" = 31.5
  dimension "d60" = 5.5
  dimension "d61" = 6.5
  dimension "d62" = 31.5
  dimension "d63" = 5.5
  dimension "d64" = 31.5
  dimension "d65" = 5.5
  dimension "d66" = 31.5
  dimension "d67" = 100
  dimension "d68" = 100
  dimension "d69" = 5.5
  dimension "d70" = 31.5
  dimension "d71" = 3
  dimension "d73" = 3
  dimension "d74" = 3
  dimension "d75" = 3
  dimension "d76" = 3
  dimension "d77" = 3
  dimension "d78" = 3
  dimension "d81" = 31.5
  dimension "d83" = 3
  dimension "d88" = 6.5
  dimension "d89" = 6.5
  dimension "d90" = 6.5
  dimension "d91" = 6.5
  dimension "d92" = 6.5
  dimension "d93" = 6.5
  dimension "d94" = 6.5
  dimension "d95" = 6.5
  constraint horizontal L0
  constraint vertical L1
  constraint horizontal L2
  constraint vertical L3
  constraint coincident L1.end L2.start
  constraint horizontal L4
  constraint vertical L5
  constraint horizontal L6
  constraint vertical L7
  constraint horizontal L8
  constraint vertical L9
  constraint horizontal L10
  constraint vertical L11
  constraint horizontal L12
  constraint vertical L13
  constraint horizontal L14
  constraint vertical L15
  constraint horizontal L16
  constraint vertical L17
  constraint horizontal L18
  constraint vertical L19
  constraint horizontal L20
  constraint vertical L21
  constraint horizontal L22
  constraint vertical L23
  constraint horizontal L24
  constraint vertical L25
  constraint horizontal L26
  constraint vertical L27
  constraint horizontal L28
  constraint vertical L29
  constraint horizontal L30
  constraint vertical L31
  constraint horizontal L32
  constraint vertical L33
  constraint midpoint L5 A0.centre
  constraint midpoint L32 A1.centre
  constraint midpoint L27 A2.centre
  constraint midpoint L23 A3.centre
  constraint midpoint L20 A4.centre
  constraint midpoint L12 A5.centre
  constraint midpoint L15 A6.centre
  constraint horizontal L34
  constraint vertical L35
  constraint horizontal L36
  constraint vertical L37
  constraint midpoint L34 A7.centre
  constraint horizontal L38
  constraint vertical L39
  constraint horizontal L40
  constraint vertical L41
  constraint horizontal L42
  constraint vertical L43
  constraint horizontal L44
  constraint vertical L45
  constraint horizontal L46
  constraint vertical L47
  constraint horizontal L48
  constraint vertical L49
  constraint horizontal L50
  constraint vertical L51
  constraint horizontal L52
  constraint vertical L53
  measures "d53" distance of L0.start L4.end
  measures "d54" distance of L0.start L6.end
  measures "d55" distance of L0.start L8.end
  measures "d57" distance of L0.end L10.end
  measures "d58" distance of L0.end L12.end
  measures "d59" distance of L0.end L14.end
  measures "d60" distance of L0.end L16.end
  measures "d61" distance of L1.end L18.end
  measures "d62" distance of L1.end L20.end
  measures "d63" distance of L1.end L24.end
  measures "d64" distance of L2.end L26.end
  measures "d65" distance of L2.end L30.end
  measures "d66" distance of L2.end L32.end
  measures "d67" distance of L3 L13
  measures "d68" distance of L0 L2
  measures "d69" distance of L26 L28
  measures "d70" distance of L23 L25
  measures "d71" diameter of A0
  measures "d73" diameter of A1
  measures "d74" diameter of A2
  measures "d75" diameter of A3
  measures "d76" diameter of A4
  measures "d77" diameter of A5
  measures "d78" diameter of A6
  measures "d81" distance of L8 L34
  measures "d83" diameter of A7
  measures "d88" distance of L0.start L8.end
  measures "d89" distance of L0.start L40.end
  measures "d90" distance of L2.end L42.end
  measures "d91" distance of L2.end L44.end
  measures "d92" distance of L1.end L18.end
  measures "d93" distance of L1.end L48.end
  measures "d94" distance of L0.end L10.end
  measures "d95" distance of L0.end L52.end
extrude "Extrude9" cut sketch "Sketch2" against normal blind 20 contours L5 A0 | L5 A0 | L15 A6 | L15 A6 | L34 A7 | L34 A7 | L32 A1 | L32 A1 | L12 A5 | L12 A5 | L20 A4 | L20 A4 | L27 A2 | L27 A2 | L23 A3 | L23 A3
extrude "Extrude10" cut sketch "Sketch2" against normal blind 3 contours L0 L3 L4 L6 L7 L8 L9 L35 L36 L37 L38 L39 L41 | L0 L4 L5 L6 L9 A0 L37 L39 | L3 L6 L9 L35 L37 L39 L40 L41 | L0 L1 L2 L3 L5 L6 L9 L11 L12 L15 L16 L19 L20 L23 L24 L27 L28 L31 L32 A0 A1 A2 A3 A4 A5 A6 L34 L37 A7 L39 L43 L44 L47 L51 | L3 L9 L34 L35 L37 A7 L40 | L0 L11 L14 L15 L16 A6 L51 | L0 L1 L10 L11 L13 L14 L16 L17 L50 L51 L53 | L3 L31 L32 L33 A1 L44 | L1 L11 L13 L16 L51 L52 L53 | L3 L28 L31 L33 L44 L45 | L1 L11 L12 L13 A5 L52 | L2 L3 L26 L28 L29 L30 L31 L33 L42 L45 | L28 L31 L43 L44 | L2 L26 L28 L31 L42 L43 | L2 L26 L27 L28 A2 L43 | L1 L19 L20 L21 A4 L48 | L1 L19 L21 L24 L47 L48 L49 | L1 L2 L18 L19 L21 L22 L24 L25 L46 L47 L49 | L2 L19 L22 L23 L24 A3 L47
extrude "Extrude11" cut sketch "Sketch2" against normal blind 70 contours L0 L3 L4 L6 L7 L8 L9 L35 L36 L37 L38 L39 L41 | L3 L6 L9 L35 L37 L39 L40 L41 | L0 L1 L10 L11 L13 L14 L16 L17 L50 L51 L53 | L1 L11 L13 L16 L51 L52 L53 | L3 L28 L31 L33 L44 L45 | L2 L3 L26 L28 L29 L30 L31 L33 L42 L45 | L28 L31 L43 L44 | L2 L26 L28 L31 L42 L43 | L1 L19 L21 L24 L47 L48 L49 | L1 L2 L18 L19 L21 L22 L24 L25 L46 L47 L49
